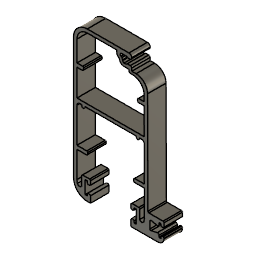
Mosquitero (Autodesk Fusion 360 design; units mm, degrees)
part number: 2025-12-27-23-45-21-865
Autodesk Fusion 360 part; units mm, degrees
note: some values were not read from the file. Set by a fixed rule: which sketch regions a step uses.
sketch "Boceto2" plane through (0, 0, 0) normal (0, 1, 0) x (1, 0, 0)
  line L0 (7.5, 0) -> (9.2213, 0)
  line L1 (0, -73.2) -> (0, -7.5)
  arc A0 (0, -73.2) -> (7.5, -80.7) centre (7.5, -73.2) ccw
  arc A1 (7.5, 0) -> (0, -7.5) centre (7.5, -7.5) ccw
  arc A2 (1.9172, -73.2) -> (7.5, -78.7828) centre (7.5, -73.2) ccw
  line L2 (7.5, -3.5523) -> (7.5, -2.6)
  line L3 (7.5, -2.6) -> (6.3, -2.6)
  line L4 (6.3, -2.6) -> (6.3, -9.6)
  line L5 (6.3, -9.6) -> (7.5, -9.6)
  line L6 (7.5, -9.6) -> (7.5, -8.5)
  line L7 (9.2213, -8.5) -> (9.2213, -10.6)
  line L8 (8.7213, -11.1) -> (4.9, -11.1)
  line L9 (4.4, -10.6) -> (4.4, -5.7)
  arc A3 (4.4, -5.7) -> (2.8546, -5.0381) centre (3.3076, -6.1153) ccw
  arc A4 (4.4, -5.7) -> (2.1854, -5.7893) centre (3.3076, -6.1153) ccw
  arc A5 (2.1854, -5.7893) -> (1.9172, -7.5) centre (7.5062, -7.5) ccw
  arc A6 (9.2213, -8.5) -> (7.5, -8.5) centre (8.3607, -9.2707) ccw
  arc A7 (7.5, -3.5523) -> (9.2213, -3.5523) centre (8.3607, -3.072) ccw
  line L10 (9.2213, -3.5523) -> (9.2213, 0)
  line L11 (20.1126, -1.9172) -> (20.115, -1.9172)
  line L12 (1.9172, -21.6025) -> (7.2, -21.6025)
  line L13 (7.7, -22.1025) -> (7.7, -23)
  line L14 (7.2, -23.5) -> (1.9172, -23.5)
  line L15 (20.0634, -43.7426) -> (20.0634, -43.7426)
  line L16 (20.036, -60.0002) -> (20.036, -60.0234)
  line L17 (1.9172, -21.6025) -> (1.9172, -7.5)
  arc A8 (7.2, -23.5) -> (7.7, -23) centre (7.2, -23) ccw
  arc A9 (7.7, -22.1025) -> (7.2, -21.6025) centre (7.2, -22.1025) ccw
  line L18 (1.9172, -42.2426) -> (1.9172, -23.5)
  arc A10 (1.9172, -42.2426) -> (3.4172, -43.7426) centre (3.4172, -42.2426) ccw
  line L19 (6.2895, -43.7426) -> (6.2895, -43.415)
  line L20 (4.4317, -43.415) -> (4.4317, -43.7426)
  arc A11 (6.2895, -43.415) -> (4.4317, -43.415) centre (5.3606, -43.415) ccw
  line L21 (20.0634, -43.7426) -> (20.0591, -43.7426)
  line L22 (4.4317, -43.7426) -> (3.4172, -43.7426)
  line L23 (1.9172, -60.0002) -> (1.9172, -45.6046)
  arc A12 (4.4, -10.6) -> (4.9, -11.1) centre (4.9, -10.6) ccw
  arc A13 (8.7213, -11.1) -> (9.2213, -10.6) centre (8.7213, -10.6) ccw
  line L24 (32.4735, -22.1342) -> (32.4712, -23.0317)
  line L25 (35.8029, -10.6401) -> (35.8154, -5.7401)
  arc A14 (36.701, -43.7851) -> (38.2048, -42.289) centre (36.7048, -42.2851) ccw
  line L26 (38.1594, -60.0465) -> (38.1962, -45.651)
  line L27 (33.8286, -43.7778) -> (33.8295, -43.4502)
  arc A15 (35.6873, -43.4549) -> (33.8295, -43.4502) centre (34.7584, -43.4526) ccw
  line L28 (32.7209, -3.5846) -> (32.7233, -2.6322)
  line L29 (35.6864, -43.7825) -> (36.701, -43.7851)
  line L30 (32.9699, -23.5329) -> (38.2527, -23.5464)
  line L31 (40.0597, -66.6685) -> (40.2, -11.7476)
  line L32 (38.2048, -42.289) -> (38.2527, -23.5464)
  arc A16 (32.4712, -23.0317) -> (32.9699, -23.5329) centre (32.9712, -23.0329) ccw
  line L33 (35.6873, -43.4549) -> (35.6864, -43.7825)
  arc A17 (37.3625, -5.0822) -> (35.8154, -5.7401) centre (36.9067, -6.1583) ccw
  line L34 (30.9869, -8.5278) -> (30.9816, -10.6278)
  arc A18 (38.2936, -7.5465) -> (38.0298, -5.8351) centre (32.7046, -7.5322) ccw
  arc A19 (35.3016, -11.1388) -> (35.8029, -10.6401) centre (35.3029, -10.6388) ccw
  arc A20 (32.9748, -21.6355) -> (32.4735, -22.1342) centre (32.9735, -22.1355) ccw
  line L35 (32.7054, -9.6322) -> (32.7082, -8.5322)
  arc A21 (30.9816, -10.6278) -> (31.4803, -11.1291) centre (31.4816, -10.6291) ccw
  line L36 (33.9233, -2.6353) -> (33.9054, -9.6353)
  arc A22 (38.0298, -5.8351) -> (35.8154, -5.7401) centre (36.9067, -6.1583) ccw
  arc A23 (30.9996, -3.5802) -> (32.7209, -3.5846) centre (31.8615, -3.102) ccw
  line L37 (30.9996, -3.5802) -> (31.0086, -0.0278)
  line L38 (38.2576, -21.649) -> (38.2936, -7.5465)
  line L39 (31.4803, -11.1291) -> (35.3016, -11.1388)
  line L40 (32.7233, -2.6322) -> (33.9233, -2.6353)
  line L41 (33.9054, -9.6353) -> (32.7054, -9.6322)
  arc A24 (32.7082, -8.5322) -> (30.9869, -8.5278) centre (31.8456, -9.3007) ccw
  line L42 (38.2576, -21.649) -> (32.9748, -21.6355)
  line L43 (20.0548, -43.7426) -> (20.0634, -43.7426)
  line L44 (20.036, -60.0234) -> (20.0383, -60.0234)
  line L45 (20.036, -61.8138) -> (20.0119, -80.7) construction
  line L46 (20.115, 0) -> (20.0591, -43.7426) construction
  line L47 (20.0567, -45.6046) -> (20.0383, -60.0234) construction
  line L48 (40.7013, -11.2489) -> (48.4387, -11.2687)
  line L49 (47.079, -9.4756) -> (46.4145, -9.4739)
  line L50 (46.215, -9.2734) -> (46.2173, -8.3924)
  line L51 (45.3178, -7.6556) -> (41.9018, -8.3505)
  line L52 (41.3021, -7.8592) -> (41.3119, -4.0405)
  line L53 (41.9227, -3.5543) -> (45.3008, -4.3224)
  line L54 (46.2171, -3.5911) -> (46.2171, -2.7085)
  line L55 (46.4176, -2.5085) -> (47.0812, -2.5102)
  line L56 (47.2807, -2.7103) -> (47.2802, -3.4742)
  line L57 (47.779, -3.9745) -> (48.4444, -3.9762)
  line L58 (48.9457, -3.4775) -> (48.9461, -3.3054)
  line L59 (31.0086, -0.0278) -> (45.7004, -0.0471)
  arc A25 (48.9461, -3.3054) -> (45.7004, -0.0471) centre (45.6961, -3.2971) ccw
  arc A26 (46.2173, -8.3924) -> (45.3178, -7.6556) centre (45.4673, -8.3905) ccw
  arc A27 (45.3008, -4.3224) -> (46.2171, -3.5911) centre (45.4671, -3.5911) ccw
  arc A28 (41.3021, -7.8592) -> (41.9018, -8.3505) centre (41.8021, -7.8605) ccw
  arc A29 (41.9227, -3.5543) -> (41.3119, -4.0405) centre (41.8119, -4.0418) ccw
  arc A30 (47.079, -9.4756) -> (47.2795, -9.2761) centre (47.0795, -9.2756) ccw
  arc A31 (47.2807, -2.7103) -> (47.0812, -2.5102) centre (47.0807, -2.7102) ccw
  arc A32 (46.4176, -2.5085) -> (46.2171, -2.7085) centre (46.4171, -2.7085) ccw
  arc A33 (46.215, -9.2734) -> (46.4145, -9.4739) centre (46.415, -9.2739) ccw
  line L60 (48.94, -10.7675) -> (48.9349, -8.6538)
  line L61 (48.4353, -8.155) -> (47.78, -8.1546)
  line L62 (47.2797, -8.6544) -> (47.2795, -9.2761)
  arc A34 (47.78, -8.1546) -> (47.2797, -8.6544) centre (47.7797, -8.6546) ccw
  arc A35 (48.9349, -8.6538) -> (48.4353, -8.155) centre (48.4349, -8.655) ccw
  arc A36 (47.2802, -3.4742) -> (47.779, -3.9745) centre (47.7802, -3.4745) ccw
  arc A37 (48.4444, -3.9762) -> (48.9457, -3.4775) centre (48.4457, -3.4762) ccw
  arc A38 (48.4387, -11.2687) -> (48.94, -10.7675) centre (48.44, -10.7687) ccw
  arc A39 (40.7013, -11.2489) -> (40.2, -11.7476) centre (40.7, -11.7489) ccw
  line L63 (1.9172, -60.0002) -> (5, -60.0002)
  line L64 (5.5, -60.5002) -> (5.5, -61.5)
  line L65 (5, -62) -> (1.9172, -62)
  line L66 (1.9172, -62) -> (1.9172, -73.2)
  arc A40 (5, -62) -> (5.5, -61.5) centre (5, -61.5) ccw
  arc A41 (5.5, -60.5002) -> (5, -60.0002) centre (5, -60.5002) ccw
  line L67 (35.0715, -62.0384) -> (38.1543, -62.0463)
  arc A42 (34.5728, -61.5371) -> (35.0715, -62.0384) centre (35.0728, -61.5384) ccw
  line L68 (34.5753, -60.5374) -> (34.5728, -61.5371)
  arc A43 (35.0766, -60.0387) -> (34.5753, -60.5374) centre (35.0753, -60.5387) ccw
  line L69 (38.1594, -60.0465) -> (35.0766, -60.0387)
  line L70 (30.75, -71.501) -> (31.8964, -71.5024)
  line L71 (38.1543, -65.2524) -> (38.1543, -62.0463)
  arc A44 (31.8964, -71.5024) -> (38.1543, -65.2524) centre (31.9043, -65.2524) ccw
  line L72 (29.999, -72.25) -> (29.9981, -73.0126)
  line L73 (23.3899, -78.7828) -> (7.5, -78.7828)
  line L74 (23.3899, -78.7828) -> (23.3899, -77.5018)
  line L75 (24.7696, -75.5018) -> (24.7696, -75.5018)
  line L76 (24.7696, -75.5018) -> (24.7696, -75.506)
  line L77 (27.2726, -73.0092) -> (29.9981, -73.0126)
  line L78 (7.5, -80.7) -> (29.9799, -80.7275)
  line L79 (31.4817, -79.2293) -> (31.4822, -78.7914)
  line L80 (30.7342, -78.0405) -> (29.2174, -78.0367)
  line L81 (28.9667, -78.286) -> (28.9668, -78.2539)
  line L82 (28.7168, -78.5033) -> (25.9982, -78.5033)
  line L83 (26.1638, -76.6384) -> (26.5435, -75.8096)
  line L84 (26.6162, -75.4764) -> (26.6162, -75.4604)
  line L85 (27.3662, -74.7104) -> (28.5562, -74.7104)
  line L86 (28.8062, -74.9604) -> (28.8062, -74.931)
  line L87 (29.0559, -75.181) -> (30.7317, -75.183)
  line L88 (31.4826, -74.4325) -> (31.4815, -72.8966)
  line L89 (31.4815, -72.8966) -> (33.7937, -72.9025)
  arc A45 (33.7937, -72.9025) -> (40.0597, -66.6685) centre (33.8097, -66.6526) ccw
  arc A46 (30.75, -71.501) -> (29.999, -72.25) centre (30.749, -72.251) ccw
  arc A47 (30.7317, -75.183) -> (31.4826, -74.4325) centre (30.7326, -74.433) ccw
  arc A48 (27.2726, -73.0092) -> (24.7696, -75.506) centre (27.2696, -75.5092) ccw
  arc A49 (24.7074, -75.6218) -> (23.3899, -77.5018) centre (25.3899, -77.5018) ccw
  arc A50 (24.7074, -75.6218) -> (24.7696, -75.506) centre (24.6304, -75.5059) ccw
  arc A51 (25.7261, -77.051) -> (25.9982, -78.5033) centre (25.9982, -77.7517) ccw
  arc A52 (27.3662, -74.7104) -> (26.6162, -75.4604) centre (27.3662, -75.4604) ccw
  arc A53 (25.7261, -77.051) -> (26.1638, -76.6384) centre (25.4365, -76.3052) ccw
  arc A54 (26.5435, -75.8096) -> (26.6162, -75.4764) centre (25.8162, -75.4764) ccw
  arc A55 (29.9799, -80.7275) -> (31.4817, -79.2293) centre (29.9817, -79.2275) ccw
  arc A56 (31.4822, -78.7914) -> (30.7342, -78.0405) centre (30.7322, -78.7905) ccw
  arc A57 (29.2174, -78.0367) -> (28.9667, -78.286) centre (29.2167, -78.2867) ccw
  arc A58 (28.7168, -78.5033) -> (28.9668, -78.2539) centre (28.7168, -78.2533) ccw
  arc A59 (28.8062, -74.931) -> (29.0559, -75.181) centre (29.0562, -74.931) ccw
  arc A60 (28.8062, -74.9604) -> (28.5562, -74.7104) centre (28.5562, -74.9604) ccw
  line L90 (1.9172, -45.6046) -> (38.1962, -45.651)
  line L91 (6.2895, -43.7426) -> (33.8286, -43.7778)
  point P0 (0, -80.7)
  point P1 (40.2299, -0.0514)
  point P2 (40.2299, -0.0514)
  dimension "d10" = 80.7
  dimension "d12" = 7.5
  dimension "d14" = 0.5
  dimension "d15" = 1.5
  dimension "d17" = 0.5
  dimension "d22" = 3.25
  dimension "d23" = 0.75
  dimension "d24" = 0.5
  dimension "d25" = 0.2
  dimension "d26" = 0.5
  dimension "d27" = 0.5
  dimension "d28" = 6.25
  dimension "d29" = 6.25
  dimension "d30" = 0.75
  dimension "d31" = 2.5
  dimension "d32" = 2
  dimension "d33" = 0.75
  dimension "d34" = 0.8
  dimension "d35" = 1.5
  dimension "d36" = 0.75
  dimension "d37" = 0.25
  constraint horizontal L0
  constraint vertical L1
  constraint coincident P0 L1
  constraint tangent L1 A0
  constraint coincident origin L0
  constraint coincident origin L1
  constraint tangent L0 A1
  constraint tangent L1 A1
  constraint equal A0 A1
  constraint perpendicular L2 L3
  constraint perpendicular L2 L5
  constraint perpendicular L5 L6
  constraint perpendicular L3 L7
  constraint perpendicular L7 L8
  constraint perpendicular L8 L9
  constraint concentric A0 A2
  constraint concentric A3 A4
  constraint coincident L11.start L46
  constraint horizontal L12
  constraint vertical L13
  constraint horizontal L14
  constraint vertical L15
  constraint horizontal L21
  constraint vertical L16
  constraint coincident L45.start L46
  constraint tangent L13 A8
  constraint tangent L14 A8
  constraint tangent L12 A9
  constraint tangent L13 A9
  constraint equal A8 A9
  constraint tangent A10 L21
  constraint tangent L18 A10
  constraint vertical L19
  constraint vertical L20
  constraint coincident L20.end L21
  constraint collinear L21 L22
  constraint tangent L8 A12
  constraint tangent L9 A12
  constraint tangent L7 A13
  constraint tangent L8 A13
  constraint equal A12 A13
  constraint symmetric origin P2 L46
  constraint symmetric A5.end A18.start L46
  constraint symmetric A7.end A23.start L46
  constraint symmetric L2.start L28.start L46
  constraint symmetric L2.end L28.end L46
  constraint symmetric L3.end L36.start L46
  constraint symmetric L4.end L36.end L46
  constraint symmetric L5.end L35.start L46
  constraint symmetric L6.end L35.end L46
  constraint symmetric L7.start L34.start L46
  constraint symmetric L9.end L25.end L46
  constraint symmetric A3 A17 L46
  constraint symmetric A3.end A17.start L46
  constraint symmetric A4 A22 L46
  constraint symmetric A4.end A18.end L46
  constraint symmetric A5 A18 L46
  constraint symmetric A6 A24 L46
  constraint symmetric A7 A23 L46
  constraint symmetric L0.end L37.end L46
  constraint symmetric L12.start L38.start L46
  constraint symmetric L14.end L30.end L46
  constraint symmetric L23.end L26.end L46
  constraint symmetric L15.start L43.start L46
  constraint symmetric L23.start L26.start L46
  constraint symmetric L13.end L24.end L46
  constraint symmetric L14.start L30.start L46
  constraint symmetric A8 A16 L46
  constraint symmetric L12.end A20.start L46
  constraint symmetric L13.start L24.start L46
  constraint symmetric A9 A20 L46
  constraint symmetric A10.end A14.start L46
  constraint symmetric L18.start A14.end L46
  constraint symmetric A10 A14 L46
  constraint symmetric L20.end L29.start L46
  constraint symmetric L19.start L27.start L46
  constraint symmetric L19.end L27.end L46
  constraint symmetric L20.start A15.start L46
  constraint symmetric A11 A15 L46
  constraint symmetric L8.end A19.start L46
  constraint symmetric L9.start L25.start L46
  constraint symmetric A12 A19 L46
  constraint symmetric L7.end L34.end L46
  constraint symmetric L8.start A21.end L46
  constraint symmetric A13 A21 L46
  constraint collinear L45 L46
  constraint collinear L46 L47
  constraint perpendicular L31 L48
  constraint perpendicular L31 L49
  constraint perpendicular L49 L50
  constraint parallel L31 L52
  constraint tangent L58 A25
  constraint tangent L59 A25
  constraint tangent L50 A26
  constraint tangent L51 A26
  constraint tangent L53 A27
  constraint tangent L54 A27
  constraint equal A26 A27
  constraint tangent L51 A28
  constraint tangent L52 A28
  constraint tangent L52 A29
  constraint tangent L53 A29
  constraint equal A28 A29
  constraint tangent L49 A30
  constraint tangent L55 A31
  constraint tangent L56 A31
  constraint equal A30 A31
  constraint tangent L54 A32
  constraint tangent L55 A32
  constraint equal A30 A32
  constraint tangent L49 A33
  constraint tangent L50 A33
  constraint equal A30 A33
  constraint perpendicular L56 L61
  constraint tangent L61 A34
  constraint tangent L62 A34
  constraint tangent L60 A35
  constraint tangent L61 A35
  constraint equal A34 A35
  constraint tangent L56 A36
  constraint tangent L57 A36
  constraint equal A34 A36
  constraint tangent L57 A37
  constraint tangent L58 A37
  constraint equal A34 A37
  constraint tangent L48 A38
  constraint tangent L60 A38
  constraint equal A34 A38
  constraint tangent L48 A39
  constraint tangent L31 A39
  constraint equal A34 A39
  constraint perpendicular L23 L63
  constraint perpendicular L63 L64
  constraint perpendicular L23 L65
  constraint tangent A2 L66
  constraint tangent L64 A40
  constraint tangent L65 A40
  constraint tangent L63 A41
  constraint tangent L64 A41
  constraint equal A40 A41
  constraint symmetric L23.start L45 L26.start
  constraint symmetric L45 L65.end L67.end
  constraint symmetric L45 L64.end A42.start
  constraint symmetric L45 L65.start L67.start
  constraint symmetric L45 A40 A42
  constraint symmetric L45 L63.end A43.start
  constraint symmetric L45 L64.start L68.start
  constraint symmetric L45 A41 A43
  constraint perpendicular L45 L70
  constraint vertical L71
  constraint tangent L70 A44
  constraint tangent L71 A44
  constraint perpendicular L70 L72
  constraint tangent A2 L73
  constraint perpendicular L73 L74
  constraint perpendicular L45 L75
  constraint parallel L77 L78
  constraint perpendicular L78 L79
  constraint perpendicular L31 L80
  constraint perpendicular L80 L81
  constraint perpendicular L82 L84
  constraint perpendicular L85 L86
  constraint perpendicular L79 L87
  constraint perpendicular L31 L89
  constraint tangent L89 A45
  constraint tangent L31 A45
  constraint tangent L70 A46
  constraint tangent L72 A46
  constraint tangent L87 A47
  constraint tangent L88 A47
  constraint equal A46 A47
  constraint tangent L76 A48
  constraint tangent L77 A48
  constraint tangent L74 A49
  constraint tangent L75 A49
  constraint tangent L76 A50
  constraint tangent L84 A52
  constraint tangent L85 A52
  constraint tangent L83 A53
  constraint tangent A51 A53
  constraint tangent L83 A54
  constraint tangent L84 A54
  constraint equal A53 A54
  constraint tangent L78 A55
  constraint tangent L79 A55
  constraint tangent L79 A56
  constraint tangent L80 A56
  constraint tangent L80 A57
  constraint tangent L81 A57
  constraint tangent L81 A58
  constraint tangent L82 A58
  constraint equal A57 A58
  constraint tangent L86 A59
  constraint tangent L87 A59
  constraint equal A57 A59
  constraint tangent L85 A60
  constraint tangent L86 A60
  constraint equal A57 A60
  measures "d10" distance of origin P0
  measures "d12" radius of A0
  measures "d14" radius of A8
  measures "d15" radius of A10
  measures "d17" radius of A12
  measures "d22" radius of A25
  measures "d23" radius of A26
  measures "d24" radius of A28
  measures "d25" radius of A30
  measures "d26" radius of A34
  measures "d27" radius of A40
  measures "d28" radius of A44
  measures "d29" radius of A45
  measures "d30" radius of A46
  measures "d31" radius of A48
  measures "d32" radius of A49
  measures "d33" radius of A52
  measures "d34" radius of A53
  measures "d35" radius of A55
  measures "d36" radius of A56
  measures "d37" radius of A57
extrude "Extruir1" add sketch "Boceto2" along normal blind 10
equation "d19 = L"
equation "L = 10 mm"
